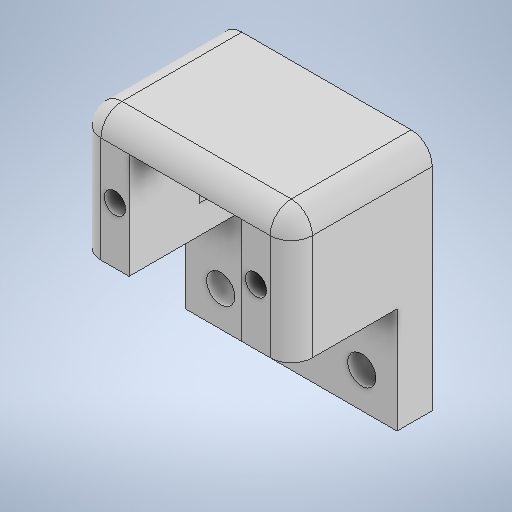
# Autodesk Inventor part: IR_bracket
Saved by Autodesk Inventor 2026.1 (Build 301233000, 233)
## iProperties
Created: 2026-05-21
Part Number: IR_bracket
Material: Generic
Document SubType Name: Modeling
Designer: chris
Density: 1 g/cm^3
Appearance: Default
Author: chris
Autodesk Inventor part; units mm, degrees
ref_plane "YZ Plane" through (0, 0, 0) normal (1, 0, 0) x (0, 1, 0)
ref_plane "XZ Plane" through (0, 0, 0) normal (0, 1, 0) x (-1, 0, 0)
ref_plane "XY Plane" through (0, 0, 0) normal (0, 0, 1) x (1, 0, 0)
sketch "Sketch1" plane through (0, 0, 0) normal (0, 0, 1) x (1, 0, 0)
  line L0 (-15, -10) -> (15, -10)
  line L1 (15, -10) -> (15, 10)
  line L2 (15, 10) -> (-15, 10)
  line L3 (-15, 10) -> (-15, -10)
  line L4 (-15, -10) -> (15, 10) construction
  line L5 (15, -10) -> (-15, 10) construction
  point P0 (0, 0)
  dimension "d0" = 30
  dimension "d1" = 20
  constraints: 12 end point, 2 midpoint, 2 parallel, 1 horizontal, 1 perpendicular
  measures "d0" distance of L2.end L1.end
  measures "d1" distance of L0.end L1.end
extrude "Extrusion1" add sketch "Sketch1" against normal blind 5
sketch "Sketch2" plane through (0, 0, 0) normal (0, 0, 1) x (1, 0, 0)
  line L0 (-15, 0) -> (15, 0)
  line L1 (15, 0) -> (15, 15)
  line L2 (15, 15) -> (-15, 15)
  line L3 (-15, 15) -> (-15, 0)
  line L4 (-15, 0) -> (15, 15) construction
  line L5 (15, 0) -> (-15, 15) construction
  line L6 (15, 10) -> (-15, 10) projected
  line L7 (-15, 10) -> (-15, -10) projected
  point P0 (0, 0)
  point P1 (0, 7.5)
  dimension "d4" = 30
  dimension "d5" = 15
  dimension "d18" = 5
  constraints: 12 end point, 2 midpoint, 2 parallel, 1 collinear, 1 horizontal, 1 perpendicular, 1 other
  measures "d4" distance of L1.end L2.end
  measures "d5" distance of L0.end L1.end
extrude "Extrusion2" add sketch "Sketch2" along normal blind 15
sketch "Sketch3" plane through (0, 0, 0) normal (0, 0, 1) x (1, 0, 0)
  circle A0 centre (10, -10) radius 2
  circle A1 centre (-10, -10) radius 2
  line L0 (-15, -10) -> (15, -10) projected
  line L1 (-15, 0) -> (-15, -10) projected
  point P0 (0, 0)
  dimension "d8" = 4
  dimension "d9" = 4
  dimension "d12" = 5
  dimension "d13" = 20
  constraints: 2 centre point, 2 point on line
  measures "d8" diameter of A1
  measures "d9" diameter of A0
  measures "d12" distance from line of L1 A1.centre
  measures "d13" distance of A1.centre A0.centre
sketch "Sketch4" plane through (-15, -10, 0) normal (0, -1, 0) x (1, 0, 0)
  line L0 (0, -5) -> (30, -5)
  line L1 (30, -5) -> (30, 0)
  line L2 (30, 0) -> (0, 0)
  line L3 (0, 0) -> (0, -5)
  line L4 (0, -5) -> (30, 0) construction
  line L5 (30, -5) -> (0, 0) construction
  line L6 (0, 0) -> (30, 0) projected
  line L7 (30, 0) -> (30, -5) projected
  line L8 (0, 0) -> (0, -5) projected
  line L9 (30, -5) -> (0, -5) projected
  point P0 (15, 0)
  point P1 (15, -2.5)
  constraints: 12 end point, 4 collinear, 2 midpoint, 2 parallel, 1 horizontal, 1 perpendicular
extrude "Extrusion3" add sketch "Sketch4" along normal blind 5
extrude "Extrusion4" cut sketch "Sketch3" against normal blind 5
sketch "Sketch5" plane through (0, 0, -5) normal (0, 0, -1) x (-1, 0, 0)
  line L0 (-8, 0) -> (8, 0)
  line L1 (8, 0) -> (8, 15)
  line L2 (8, 15) -> (-8, 15)
  line L3 (-8, 15) -> (-8, 0)
  line L4 (-8, 0) -> (8, 15) construction
  line L5 (8, 0) -> (-8, 15) construction
  line L6 (-15, 15) -> (15, 15) projected
  point P0 (0, 0)
  point P1 (0, 7.5)
  dimension "d16" = 16
  dimension "d21" = 15
  dimension "d22" = 0
  constraints: 12 end point, 2 midpoint, 2 parallel, 1 horizontal, 1 perpendicular
  measures "d16" distance of L2.end L1.end
  measures "d21" distance of L0.end L1.end
  measures "d22" distance between parallel lines of L6 L2
sketch "Sketch6" plane through (0, 0, 0) normal (0, 0, -1) x (-1, 0, 0)
  line L0 (-15, 10) -> (15, 10)
  line L1 (15, 10) -> (15, 15)
  line L2 (15, 15) -> (-15, 15)
  line L3 (-15, 15) -> (-15, 10)
  line L4 (-15, 10) -> (15, 15) construction
  line L5 (15, 10) -> (-15, 15) construction
  line L6 (-15, 15) -> (15, 15) projected
  line L7 (15, 10) -> (-15, 10) projected
  line L8 (-15, 10) -> (-15, 15) projected
  line L9 (15, 15) -> (15, 10) projected
  point P0 (0, 0)
  point P1 (0, 12.5)
  constraints: 12 end point, 4 collinear, 2 midpoint, 2 parallel, 1 horizontal, 1 perpendicular
extrude "Extrusion5" add sketch "Sketch6" along normal blind 5
extrude "Extrusion6" cut sketch "Sketch5" against normal through all
sketch "Sketch7" plane through (0, 0, -5) normal (0, 0, -1) x (-1, 0, 0)
  circle A0 centre (-10, 8) radius 1.5
  circle A1 centre (10, 8) radius 1.5
  line L0 (-15, 15) -> (-15, -15) projected
  line L1 (8, 0) -> (-8, 0) projected
  point P0 (0, 0)
  dimension "d25" = 3
  dimension "d26" = 3
  dimension "d27" = 20
  dimension "d28" = 5
  dimension "d33" = 8
  constraints: 2 centre point, 1 horizontal alignment
  measures "d25" diameter of A0
  measures "d26" diameter of A1
  measures "d27" distance of A1.centre A0.centre
  measures "d28" distance from line of L0 A0.centre
  measures "d33" distance from line of L1 A0.centre
extrude "Extrusion7" cut sketch "Sketch7" against normal through all
sketch "Sketch8" plane through (15, 15, 15) normal (0, 1, 0) x (1, 0, 0)
  line L0 (0, 20) -> (-30, 20)
  line L1 (-30, 20) -> (-30, 0)
  line L2 (-30, 0) -> (0, 0)
  line L3 (0, 0) -> (0, 20)
  line L4 (0, 20) -> (-30, 0) construction
  line L5 (-30, 20) -> (0, 0) construction
  line L6 (0, 0) -> (-7, 0) projected
  line L7 (0, 0) -> (0, 20) projected
  line L8 (-23, 20) -> (-7, 20) projected
  line L9 (-30, 20) -> (-30, 0) projected
  point P0 (-15, 15)
  point P1 (-15, 10)
  constraints: 12 end point, 4 collinear, 2 midpoint, 2 parallel, 1 horizontal, 1 perpendicular
extrude "Extrusion8" add sketch "Sketch8" along normal blind 3
sketch "Sketch9" plane through (0, 0, -5) normal (0, 0, -1) x (-1, 0, 0)
  line L0 (-13, 4) -> (-8, 4)
  line L1 (-8, 4) -> (-8, 12)
  line L2 (-8, 12) -> (-13, 12)
  line L3 (-13, 12) -> (-13, 4)
  line L4 (-13, 4) -> (-8, 12) construction
  line L5 (-8, 4) -> (-13, 12) construction
  line L6 (8, 4) -> (13, 4)
  line L7 (13, 4) -> (13, 12)
  line L8 (13, 12) -> (8, 12)
  line L9 (8, 12) -> (8, 4)
  line L10 (8, 4) -> (13, 12) construction
  line L11 (13, 4) -> (8, 12) construction
  line L12 (-8, 0) -> (-8, 15) projected
  line L13 (8, 15) -> (8, 0) projected
  line L14 (8, 0) -> (-8, 0) projected
  point P0 (0, 0)
  point P1 (-10.5, 8)
  point P2 (10.5, 8)
  dimension "d34" = 5
  dimension "d35" = 5
  dimension "d36" = 8
  dimension "d37" = 8
  dimension "d38" = 8
  constraints: 24 end point, 4 midpoint, 4 parallel, 2 collinear, 2 horizontal, 2 perpendicular, 1 horizontal alignment
  measures "d34" distance of L1.end L2.end
  measures "d35" distance of L7.end L8.end
  measures "d36" distance of L2.end L0.start
  measures "d37" distance of L6.end L7.end
  measures "d38" distance from line of point (-10.5, 8) L14
extrude "Extrusion9" cut sketch "Sketch9" against normal blind 10
fillet "Fillet1" radius 3 2 edges at (15, 18, 5) (-15, 18, 5)
fillet "Fillet2" radius 3 3 edges at (15, 7.5, 15) (-15, 7.5, 15) (0, 18, 15)
body "Solid1"
